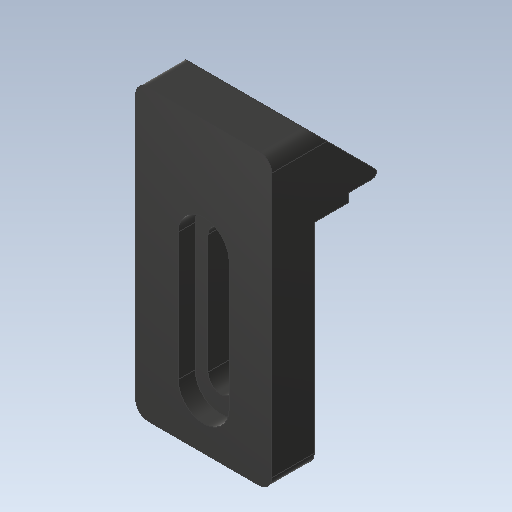
# Autodesk Inventor part: Trzymacz
Saved by Autodesk Inventor 2020 (Build 240168000, 168)
## iProperties
Created: 2019-05-26
Part Number: Trzymacz
Material: Tworzywo sztuczne ABS
Document SubType Name: Modeling
Designer: barto
Density: 1.06 g/cm^3
Appearance: Gładki —_ biały
Author: barto
Autodesk Inventor part; units mm, degrees
ref_plane "YZ Plane" through (0, 0, 0) normal (1, 0, 0) x (0, 1, 0)
ref_plane "XZ Plane" through (0, 0, 0) normal (0, 1, 0) x (-1, 0, 0)
ref_plane "XY Plane" through (0, 0, 0) normal (0, 0, 1) x (1, 0, 0)
sketch "Szkic1" plane through (0, 0, 0) normal (0, 0, 1) x (1, 0, 0)
  line L0 (-7.3846, 18.9091) -> (8.6154, 18.9091)
  line L1 (8.6154, 18.9091) -> (8.6154, -15.0909)
  line L2 (8.6154, -15.0909) -> (-7.3846, -15.0909)
  line L3 (-7.3846, -15.0909) -> (-7.3846, 18.9091)
  point P0 (0, 0)
  dimension "d1" = 16
  dimension "d2" = 34
  constraints: 8 end point, 2 parallel, 1 horizontal, 1 perpendicular
  measures "d1" distance of L0.start L0.end
  measures "d2" distance of L0.end L1.end
extrude "Wyciągnięcie proste1" add sketch "Szkic1" along normal blind 5
sketch "Szkic2" plane through (0, 0, 0) normal (0, 0, -1) x (-1, 0, 0)
  line L0 (-8.6154, 18.9091) -> (7.3846, 18.9091) projected
  line L1 (7.3846, 18.9091) -> (7.3846, -15.0909) projected
  line L2 (-8.6154, 18.9091) -> (7.3846, 18.9091)
  line L3 (7.3846, 18.9091) -> (7.3846, 9.9091)
  line L4 (7.3846, 9.9091) -> (-8.6154, 9.9091)
  line L5 (-8.6154, 9.9091) -> (-8.6154, 18.9091)
  point P0 (0, 0)
  dimension "d5" = 9
  constraints: 8 end point, 2 parallel, 1 horizontal, 1 perpendicular, 1 point on line
  measures "d5" distance of L4.end L0.start
extrude "Wyciągnięcie proste2" add sketch "Szkic2" along normal blind 8
chamfer "Faza1" distance 8 angle 45 1 edges at (0.6154, 18.9091, -8)
sketch "Szkic3" plane through (0, 0, 5) normal (0, 0, 1) x (1, 0, 0)
  line L0 (-2.3846, 8.9091) -> (3.6154, 8.9091)
  line L1 (3.6154, 8.9091) -> (3.6154, -12.0909)
  line L2 (3.6154, -12.0909) -> (-2.3846, -12.0909)
  line L3 (-2.3846, -12.0909) -> (-2.3846, 8.9091)
  line L4 (8.6154, 18.9091) -> (-7.3846, 18.9091) projected
  line L5 (-7.3846, -15.0909) -> (8.6154, -15.0909) projected
  line L6 (8.6154, -15.0909) -> (8.6154, 18.9091) projected
  point P0 (0, 0)
  dimension "d11" = 10
  dimension "d12" = 3
  dimension "d13" = 6
  dimension "d14" = 5
  constraints: 8 end point, 2 parallel, 1 horizontal, 1 perpendicular
  measures "d11" distance between parallel lines of L4 L0
  measures "d12" distance between parallel lines of L5 L2
  measures "d13" distance between parallel lines of L1 L3
  measures "d14" distance between parallel lines of L6 L1
extrude "Wyciągnięcie proste3" cut sketch "Szkic3" against normal blind 2
sketch "Szkic4" plane through (0, 0, 3) normal (0, 0, 1) x (1, 0, 0)
  line L0 (-0.8846, 6.9091) -> (2.1154, 6.9091)
  line L1 (2.1154, 6.9091) -> (2.1154, -10.0909)
  line L2 (2.1154, -10.0909) -> (-0.8846, -10.0909)
  line L3 (-0.8846, -10.0909) -> (-0.8846, 6.9091)
  line L4 (-2.3846, 8.9091) -> (3.6154, 8.9091) projected
  line L5 (3.6154, 8.9091) -> (3.6154, -12.0909) projected
  line L6 (3.6154, -12.0909) -> (-2.3846, -12.0909) projected
  point P0 (0, 0)
  dimension "d17" = 2
  dimension "d19" = 3
  dimension "d20" = 1.5
  dimension "d21" = 2
  constraints: 8 end point, 2 parallel, 1 horizontal, 1 perpendicular
  measures "d17" distance between parallel lines of L4 L0
  measures "d19" distance between parallel lines of L3 L1
  measures "d20" distance between parallel lines of L5 L1
  measures "d21" distance between parallel lines of L6 L2
extrude "Wyciągnięcie proste4" cut sketch "Szkic4" against normal up to next
fillet "Zaokrąglenie1" radius 3 4 edges at (3.6154, 8.9091, 4) (-2.3846, 8.9091, 4) (-2.3846, -12.0909, 4) (3.6154, -12.0909, 4)
fillet "Zaokrąglenie2" radius 1.5 4 edges at (-0.8846, 6.9091, 1.5) (2.1154, 6.9091, 1.5) (-0.8846, -10.0909, 1.5) (2.1154, -10.0909, 1.5)
fillet "Zaokrąglenie3" radius 1.5 4 edges at (-7.3846, -15.0909, 2.5) (8.6154, -15.0909, 2.5) (8.6154, 18.9091, 2.5) (-7.3846, 18.9091, 2.5)
sketch "Szkic5" plane through (-7.3846, 9.9091, 0) normal (0, -1, 0) x (1, 0, 0)
  line L0 (0, 0) -> (0, -8) projected
  line L1 (16, 0) -> (16, -8) projected
  line L2 (0, -8) -> (16, -8)
  line L3 (16, -8) -> (16, -4)
  line L4 (16, -4) -> (0, -4)
  line L5 (0, -4) -> (0, -8)
  line L6 (14.5, 0) -> (1.5, 0) projected
  point P0 (7.3846, 0)
  dimension "d28" = 4
  constraints: 8 end point, 2 parallel, 1 horizontal, 1 midpoint, 1 perpendicular
  measures "d28" distance between parallel lines of L6 L4
extrude "Wyciągnięcie proste5" cut sketch "Szkic5" against normal blind 1
fillet "Zaokrąglenie5" radius 0.5 1 edges at (0.6154, 10.9091, -8)
